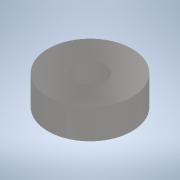
# Autodesk Inventor part: ベアリング_6-17
Saved by Autodesk Inventor 2020.3 (Build 243373000, 373)
## iProperties
Created: 2020-07-06
Part Number: ベアリング_6-17
Material: 鋼、炭素鋼
Document SubType Name: Modeling
Designer: totot
Density: 7.85 g/cm^3
Appearance: 半つや出し
Author: totot
Autodesk Inventor part; units mm, degrees
ref_plane "YZ Plane" through (0, 0, 0) normal (1, 0, 0) x (0, 1, 0)
ref_plane "XZ Plane" through (0, 0, 0) normal (0, 1, 0) x (-1, 0, 0)
ref_plane "XY Plane" through (0, 0, 0) normal (0, 0, 1) x (1, 0, 0)
sketch "スケッチ1" plane through (0, 0, 0) normal (0, 1, 0) x (-1, 0, 0)
  circle A0 centre (0, 0) radius 8.5
  circle A1 centre (0, 0) radius 3
  dimension "d0" = 17
  dimension "d1" = 6
  constraints: 2 centre point, 2 coincident
  measures "d0" diameter of A0
  measures "d1" diameter of A1
extrude "押し出し1" add sketch "スケッチ1" along normal blind 6
fillet "フィレット1" radius 0.5 4 edges at (8.5, 0, 0) (8.5, 6, 0) (3, 0, 0) (3, 6, 0)
